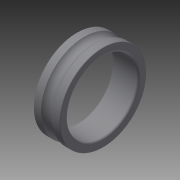
# Autodesk Inventor part: 6008_PART1
Saved by Autodesk Inventor 2014 SP2 (Build 180246200, 246)
## iProperties
Created: 2018-11-17
Part Number: 6008_PART1
Material: Generic
Catalog Web Link: www.cadenas.de
Description: -Deep groove ball bearings
Vendor: SKF
Document SubType Name: Modeling
Designer: psadmin
Manufacturer: SKF
Mass: 8.5834 g
Surface Area: 54.4501 cm^2
Volume: 8.5834 cm^3
Density: 1 g/cm^3
Appearance: PSOLRGB-175-175-175
Category: PARTsolutions
Company: SKF
Title: 6008_PART1
Author: Cadenas PARTsolutions
Comments: Deep groove ball bearings
PSOL_IDENT_0: {$CADENAS_DATA\23d-libs\skf\bearings_units_and_housings\ball_bearings\deep_groove_ball_bearings\bb1_
PSOL_IDENT_1: 001_101.prj},186 {VTYP=3D},{NB=6008_PART1},{LINA=6008_PART1},{NN=BB1_001_101_PART1},{NOPRJ=TRUE},{DA
PSOL_IDENT_2: TE=05.11.2018 07:58:23},{GEOMDATE=08.08.2018 12:16:40},{VERSION=},{LINEID=6500},{WBVAR=},{WBNUMERIC=
PSOL_IDENT_3: }  {NB=6008_PART1},{LINA=6008_PART1},{KT=DUMMY},{PRODUCTID=1050010008},{DESIGNATION=6008},{DD=40.00}
PSOL_IDENT_4: ,{D=68.000},{B=15.000},{C=0.000},{DD1=49.25},{DD2=0.0},{D1=0.00},{D2=61.10},{D3=0.00},{D4=0.000},{HH=
PSOL_IDENT_5: MIN},{BB=0.000},{FF=0.00},{R0MAX=MIN},{R0=MIN},{R12=1.10},{PITCH=54.00},{DW=7.938},{DDAMIN=44.600},{
PSOL_IDENT_6: DDAMAX=MIN},{DDBMIN=MIN},{DDBMAX=MIN},{DBMIN=MIN},{DAMAX=63.400},{BBAMIN=MIN},{CAMAX=MIN},{RAMAX=1.0
PSOL_IDENT_7: 00},{LOAD1=17.800},{LOAD2=11.000},{LOAD3=0.490},{SPEED1=22000},{SPEED2=14000},{KR=0.025},{F0=15.000}
PSOL_IDENT_8: ,{Z=12},{II=1},{MASS=0.192},{BEARING=6008},{RING=},{HELP=4.341},{HELP2=3.450},{DD1ALG=24.625},{YALG=
PSOL_IDENT_9: 24.625},{PITCH1=54.000},{DW1=7.938},{YALG1=29.659},{HALG1=4.341},{SH=24.625},{CU=1.412},{DESIGN=dgbb
PSOL_IDENT_10: 1},{HALG=4.625},{B1=0},{ALGO=1.000}
NT: Deep groove ball bearings
NB: 6008_PART1
NBSYN: $DESIGNATION._PART1
LINA: 6008_PART1
SUPPLIER: SKF
ARTICLENO: 6008_PART1
BOMINFO: 6008_PART1
CREATOR: CADENAS GmbH
Autodesk Inventor part; units mm, degrees
ref_plane "YZ Plane" through (0, 0, 0) normal (1, 0, 0) x (0, 1, 0)
ref_plane "XZ Plane" through (0, 0, 0) normal (0, 1, 0) x (-1, 0, 0)
ref_plane "XY Plane" through (0, 0, 0) normal (0, 0, 1) x (1, 0, 0)
sketch "Sketch_54" plane through (0, 0, 0) normal (0, 0, 1) x (1, 0, 0)
  line L0 (100, 0) -> (-100, 0)
  arc A0 (0, 21.1) -> (1.1, 20) centre (1.1, 21.1) ccw
  line L1 (1.1, 20) -> (13.9, 20)
  arc A1 (13.9, 20) -> (15, 21.1) centre (13.9, 21.1) ccw
  line L2 (15, 21.1) -> (15, 24.2583)
  arc A2 (15, 24.2583) -> (14.6333, 24.625) centre (14.6333, 24.2583) ccw
  line L3 (14.6333, 24.625) -> (10.68, 24.625)
  arc A3 (4.32, 24.625) -> (10.68, 24.625) centre (7.5, 27) ccw
  line L4 (4.32, 24.625) -> (0.3667, 24.625)
  arc A4 (0.3667, 24.625) -> (0, 24.2583) centre (0.3667, 24.2583) ccw
  line L5 (0, 24.2583) -> (0, 21.1)
  constraints: 12 end point, 10 point on circle, 5 centre point
revolve "Revolution1" add sketch "Sketch_54" angle 360 about axis through (100, 0, 0) along (1, 0, 0)
body "Solid1"
